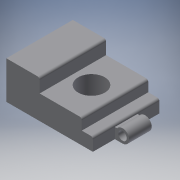
# Autodesk Inventor part: Hinge, Explosion Button
Saved by Autodesk Inventor 2016 (Build 200138000, 138)
## iProperties
Created: 2016-03-16
Part Number: Hinge, Explosion Button
Material: Generic
Document SubType Name: Modeling
Designer: Owner
Density: 1 g/cm^3
Appearance: Default
Author: Owner
Autodesk Inventor part; units mm, degrees
ref_plane "YZ Plane" through (0, 0, 0) normal (1, 0, 0) x (0, 1, 0)
sketch "Sketch1" plane through (0, 0, 0) normal (0, 0, 1) x (1, 0, 0)
  line L0 (0, 0) -> (3.81, 0)
  line L1 (0, 0) -> (0, 1.27)
  arc A0 (3.81, 0) -> (1.359061, 1.27) centre (3.81, 3) ccw
  circle A1 centre (3.81, 3) radius 1.9
  line L2 (0, 1.27) -> (1.359061, 1.27)
  dimension "d0" = 3.81
  dimension "d1" = 1.27
  dimension "d2" = 6
  dimension "d3" = 3.8
  constraints: 6 end point, 2 centre point, 2 point on circle, 1 coincident, 1 horizontal, 1 perpendicular, 1 tangent, 1 vertical
  measures "d0" distance of L0.start L0.end
  measures "d1" distance of L0.start L1.end
  measures "d2" diameter of A0
  measures "d3" diameter of A1
extrude "Extrusion1" add sketch "Sketch1" along normal blind 30.48
ref_plane "Work Plane1" through (0, 0, 20.32) normal (0, 0, 1) x (1, 0, 0)
sketch "Sketch2" plane through (0, 0, 20.32) normal (0, 0, 1) x (1, 0, 0)
  arc A0 (3.81, 0) -> (1.359061, 1.27) centre (3.81, 3) ccw
  line L0 (2.54, 1.27) -> (2.54, 0)
  line L1 (0, 0) -> (3.81, 0)
  line L2 (2.54, 0) -> (3.81, 0)
  circle A1 centre (3.81, 3) radius 0.762
  constraints: 4 end point, 1 centre point, 1 coincident, 1 horizontal, 1 point on line, 1 tangent, 1 vertical, 1 other
sketch "Sketch2 outline for Extrusion5" plane through (0, 0, 20.32) normal (0, 0, 1) x (1, 0, 0)
  line L0 (2.54, 0) -> (3.81, 0)
  line L1 (1.359061, 1.27) -> (2.54, 0)
  arc A0 (3.81, 0) -> (1.359061, 1.27) centre (3.81, 3) ccw
  circle A1 centre (3.81, 3) radius 0.762
extrude "Extrusion5" cut sketch "Sketch2 outline for Extrusion5" along normal blind 25.4
ref_plane "Work Plane3" through (0, 0, 10.16) normal (0, 0, -1) x (-1, 0, 0)
sketch "Sketch6" plane through (0, 0, 10.16) normal (0, 0, -1) x (-1, 0, 0)
  line L0 (-1.359061, 1.27) -> (-2.54, 0)
  line L1 (-1.359061, 1.27) -> (-2.54, 0)
  circle A0 centre (-3.81, 1.27) radius 0.762
  arc A1 (-1.359061, 1.27) -> (-3.81, 0) centre (-3.81, 3) ccw
  line L2 (-2.54, 0) -> (-3.81, 0)
  point P0 (0, 0)
  constraints: 4 end point, 1 centre point, 1 collinear, 1 horizontal, 1 tangent
extrude "Extrusion6" cut sketch "Sketch6" along normal blind 25.4
sketch "Sketch8" plane through (0, 0, 30.48) normal (0, 0, 1) x (1, 0, 0)
  line L0 (1.633512, 1.27) -> (1.633512, 0)
  line L1 (1.633512, 1.27) -> (1.633512, 0)
  line L2 (1.359061, 1.27) -> (2.54, 0)
  line L3 (1.633512, 0) -> (2.54, 0)
  line L4 (1.359061, 1.27) -> (0, 1.27)
  line L5 (2.54, 0) -> (1.633512, 1.27)
  point P0 (0, 0)
  constraints: 6 end point, 1 perpendicular, 1 vertical, 2 other
extrude "Extrusion8" cut sketch "Sketch8" against normal blind 10.16
sketch "Sketch9" plane through (0, 0, 0) normal (0, 0, -1) x (-1, 0, 0)
  arc A0 (-4.571927, 1.259464) -> (-3.048073, 1.259464) centre (-3.81, 1.27) ccw
  arc A1 (-4.571927, 1.259464) -> (-3.048073, 1.259464) centre (-3.81, 3) ccw
  point P0 (0, 0)
extrude "Extrusion9" cut sketch "Sketch9" against normal blind 10.16
sketch "Sketch10" plane through (0, 0, 0) normal (0, 0, -1) x (-1, 0, 0)
  line L0 (-1.359061, 1.27) -> (0, 1.27)
  line L1 (-1.359061, 1.27) -> (-1.359061, 0)
  line L2 (-1.359061, 0) -> (-2.542741, 0)
  line L3 (-2.542741, 0) -> (-1.359061, 1.27)
  point P0 (0, 0)
  constraints: 6 end point, 1 perpendicular, 1 vertical
extrude "Extrusion10" cut sketch "Sketch10" against normal blind 10.16
sketch "Sketch11" plane through (0, 0, 30.48) normal (0, 0, 1) x (1, 0, 0)
  line L0 (1.359061, 1.27) -> (1.633512, 1.27)
  line L1 (1.359061, 1.27) -> (1.633512, 0.974851)
  line L2 (1.633512, 1.27) -> (1.633512, 0.974851)
  line L3 (1.633512, 0.974851) -> (1.359061, 1.27)
  point P0 (0, 0)
  constraints: 6 end point, 1 collinear, 1 horizontal, 1 perpendicular
extrude "Extrusion11" add sketch "Sketch11" against normal blind 10.16
sketch "Sketch12" plane through (0, 1.27, 30.48) normal (0, 1, 0) x (1, 0, 0)
  line L0 (1.359061, 30.48) -> (1.359061, 20.32)
  line L1 (1.359061, 30.48) -> (-8.640939, 30.48)
  line L2 (-8.640939, 30.48) -> (-8.640939, 0)
  line L3 (-8.640939, 0) -> (1.359061, 0)
  line L4 (1.359061, 0) -> (1.359061, 30.48)
  point P0 (0, 30.48)
  dimension "d34" = 10
  constraints: 8 end point, 2 parallel, 1 horizontal, 1 perpendicular
  measures "d34" distance of L2.end L3.end
extrude "Extrusion12" add sketch "Sketch12" against normal blind 1.27
sketch "Sketch13" plane through (1.633512, 1.27, 30.48) normal (0, 1, 0) x (1, 0, 0)
  line L0 (-0.274451, 30.48) -> (-0.274451, 20.32)
  line L1 (-0.274451, 20.32) -> (-0.274451, 0)
  line L2 (-0.274451, 0) -> (1.648434, 0)
  line L3 (1.648434, 0) -> (1.648434, 10.16)
  line L4 (2.176488, 10.16) -> (0, 10.16)
  line L5 (-0.274451, 10.16) -> (1.648434, 10.16)
  point P0 (-1.633512, 30.48)
  constraints: 8 end point, 3 perpendicular, 1 midpoint, 1 point on line, 1 vertical
extrude "Extrusion13" cut sketch "Sketch13" against normal blind 1.27
sketch "Sketch14" plane through (1.359061, 0, 0) normal (1, 0, 0) x (0, 0, -1)
  line L0 (-30.474923, 6.35) -> (0.005077, 6.35)
  line L1 (0.005077, 6.35) -> (0.005077, 0)
  line L2 (0, 1.27) -> (-30.48, 1.27)
  line L3 (0, 1.27) -> (-30.474923, 1.27)
  line L4 (-30.474923, 1.27) -> (-30.474923, 5.77)
  line L5 (-30.474923, 5.77) -> (0, 5.77)
  line L6 (0, 5.77) -> (0, 1.27)
  point P0 (0, 0)
  dimension "d39" = 4.5
  constraints: 8 end point, 2 parallel, 1 horizontal, 1 perpendicular
  measures "d39" distance of L5.end L2.start
extrude "Extrusion14" add sketch "Sketch14" against normal blind 10
sketch "Sketch15" plane through (1.359061, 0, 20.32) normal (1, 0, 0) x (0, 0, -1)
  line L0 (-10.154923, 5.77) -> (20.32, 5.77)
  line L1 (20.32, 0) -> (20.07, 0)
  line L2 (20.07, 0) -> (20.07, 5.77)
  line L3 (20.07, 5.77) -> (20.32, 5.77)
  line L4 (20.32, 5.77) -> (20.32, 0)
  line L5 (-10.154923, 5.77) -> (20.32, 5.77)
  line L6 (5.082538, 5.77) -> (5.082538, 11.076995)
  line L7 (-10.154923, 0) -> (-9.904923, 0)
  line L8 (-9.904923, 0) -> (-9.904923, 5.77)
  line L9 (-10.154923, 5.77) -> (-10.154923, 0)
  line L10 (-10.154923, 0) -> (-9.904923, 0)
  line L11 (-9.904923, 0) -> (-9.904923, 5.77)
  line L12 (-9.904923, 5.77) -> (-10.154923, 5.77)
  line L13 (-10.154923, 5.77) -> (-10.154923, 0)
  dimension "d42" = 0.25
  constraints: 24 end point, 4 parallel, 4 symmetric about line, 2 horizontal, 2 perpendicular, 1 midpoint, 1 point on line, 1 vertical
  measures "d42" distance of L1.start L1.end
extrude "Extrusion15" cut sketch "Sketch15" against normal blind 10
sketch "Sketch16" plane through (1.359061, 0, 30.474923) normal (0, 0, -1) x (-1, 0, 0)
  line L0 (0, 1.27) -> (10, 1.27) projected
  line L1 (0, 0) -> (0, 1.27) projected
  line L2 (10, 0) -> (0, 0) projected
  line L3 (10, 1.27) -> (10, 0) projected
  point P0 (1.359061, 0)
extrude "Extrusion16" cut sketch "Sketch16" against normal blind 10
sketch "Sketch17" plane through (1.359061, 5.77, 30.224923) normal (0, 1, 0) x (1, 0, 0)
  line L0 (-5, 33.422895) -> (-5, -3.422186)
  line L1 (0, 29.974923) -> (-10, 29.974923)
  line L2 (-10, 0) -> (-10, 29.974923)
  line L3 (-5, 29.974923) -> (-10, 29.974923)
  line L4 (-10, 29.974923) -> (-10, 0)
  line L5 (-10, 0) -> (-5, 0)
  line L6 (-5, 0) -> (-5, 29.974923)
  point P0 (-1.359061, 30.224923)
  constraints: 8 end point, 2 parallel, 1 horizontal, 1 midpoint, 1 perpendicular
extrude "Extrusion17" add sketch "Sketch17" along normal blind 5
sketch "Sketch18" plane through (1.359061, 0, 0.25) normal (0, 0, -1) x (-1, 0, 0)
  line L0 (40, 0) -> (40, 21.034494)
  line L1 (40, 37.49) -> (40, 17.49)
  line L2 (10, 10.77) -> (5, 10.77)
  line L3 (10, 10.77) -> (40, 10.77)
  line L4 (40, 10.77) -> (40, 0)
  line L5 (40, 0) -> (10, 0)
  line L6 (10, 0) -> (10, 10.77)
  line L7 (25, 10.77) -> (40, 10.77)
  line L8 (40, 10.77) -> (40, 17.49)
  line L9 (40, 17.49) -> (25, 17.49)
  line L10 (25, 17.49) -> (25, 10.77)
  point P0 (1.359061, 0)
  constraints: 16 end point, 4 parallel, 2 horizontal, 2 perpendicular, 1 midpoint
extrude "Extrusion18" add sketch "Sketch18" against normal blind 29.975
sketch "Sketch19" plane through (1.359061, 10.77, 30.224923) normal (0, 1, 0) x (1, 0, 0)
  circle A0 centre (-16.625, 15.003923) radius 6
  circle A1 centre (-16.625, 15.003923) radius 4.85
  point P0 (-1.359061, 30.224923)
  dimension "d51" = 12
  constraints: 1 centre point
  measures "d51" diameter of A0
extrude "Extrusion19" cut sketch "Sketch19" against normal blind 29.975 contours A0 | A1
sketch "Sketch20" plane through (1.359061, 0, 30.225) normal (0, 0, 1) x (1, 0, 0)
  line L0 (-25, 17.49) -> (-25, 10.77) projected
  line L1 (-40, 0) -> (-40, 17.49) projected
  line L2 (-25, 17.49) -> (-40, 17.49)
  line L3 (-40, 17.49) -> (-40, 16.99)
  line L4 (-40, 16.99) -> (-25, 16.99)
  line L5 (-25, 16.99) -> (-25, 17.49)
  point P0 (-1.359061, 0)
  dimension "d54" = 0.5
  constraints: 8 end point, 2 parallel, 1 horizontal, 1 perpendicular, 1 point on line
  measures "d54" distance between parallel lines of L4 L2
extrude "Extrusion20" cut sketch "Sketch20" against normal blind 584.2
sketch "Sketch21" plane through (1.359061, 0, 20.32) normal (1, 0, 0) x (0, 0, -1)
  line L0 (20.07, 0) -> (20.07, 5.77)
  line L1 (-9.904923, 5.77) -> (20.07, 5.77)
  line L2 (-9.904923, 5.77) -> (-9.904923, 0)
  line L3 (0, 0) -> (-9.904923, 0)
  line L4 (0, 4.73) -> (0, 0)
  line L5 (10.16, 4.73) -> (0, 4.73)
  line L6 (10.16, 0) -> (10.16, 4.73)
  line L7 (20.07, 0) -> (10.16, 0)
  point P0 (20.32, 0)
extrude "Extrusion21" cut sketch "Sketch21" against normal blind 1
sketch "Sketch22" plane through (-3.640939, 5.77, 30.224923) normal (1, 0, 0) x (0, 0, -1)
  line L0 (0, 0) -> (0, 5)
  line L1 (0, 5) -> (29.974923, 5)
  line L2 (29.974923, 0) -> (29.974923, 5)
  line L3 (29.974923, 0) -> (0, 0)
  point P0 (30.224923, -5.77)
extrude "Extrusion22" cut sketch "Sketch22" against normal blind 1
fillet "Fillet1" radius 1 3 edges at (-23.6409, 16.99, 15.2375) (-4.6409, 10.77, 15.2375) (0.3591, 5.77, 15.2375)
sketch "Sketch23" plane through (1.359061, 0, 30.225) normal (0, 0, 1) x (1, 0, 0)
  spline S0 degree 3 poles (-15.287382, 7.562173) (-14.295298, 10.29556) (-13.653422, 13.152751) (-13.101138, 18.99204) (-13.207044, 21.960303) (-14.220005, 28.120528) (-15.237278, 31.317012) (-16.686921, 34.297861) knots -3.03465801 -3.03465801 -3.03465801 -3.03465801 -2.16997566 -2.16997566 -1.29383861 -1.29383861 -0.2991038 -0.2991038 -0.2991038 -0.2991038
  arc A0 (-25, 15.99) -> (-26, 16.99) centre (-26, 15.99) ccw
  line L0 (-26, 16.99) -> (-40, 16.99)
  line L1 (-40, 16.99) -> (-40, 0)
  line L2 (-40, 0) -> (-10, 0)
  line L3 (-10, 0) -> (-10, 10.77)
  line L4 (-10, 10.77) -> (-25, 10.77)
  line L5 (-25, 10.77) -> (-25, 15.99)
  arc A1 (-1, 4.77) -> (-2, 5.77) centre (-2, 4.77) ccw
  line L6 (-6, 5.77) -> (-2, 5.77)
  line L7 (-6, 5.77) -> (-6, 9.77)
  arc A2 (-6, 9.77) -> (-7, 10.77) centre (-7, 9.77) ccw
  line L8 (-10, 10.77) -> (-7, 10.77)
  line L9 (-10, 0) -> (-10, 10.77)
  line L10 (-1, 0) -> (-10, 0)
  line L11 (-1, 0) -> (-1, 4.77)
  point P0 (-1.359061, 0)
extrude "Extrusion23" add sketch "Sketch23" against normal blind 0.025
sketch "Sketch24" plane through (-38.640939, 0, 0.25) normal (0, 0, -1) x (-1, 0, 0)
  arc A0 (-38, 5.77) -> (-39, 4.77) centre (-38, 4.77) ccw projected
  line L0 (-39, 4.77) -> (-39, 0) projected
  line L1 (-39, 0) -> (0, 0) projected
  line L2 (0, 0) -> (0, 16.99) projected
  line L3 (0, 16.99) -> (-14, 16.99) projected
  arc A1 (-14, 16.99) -> (-15, 15.99) centre (-14, 15.99) ccw projected
  line L4 (-15, 15.99) -> (-15, 10.77) projected
  line L5 (-33, 10.77) -> (-15, 10.77) projected
  arc A2 (-33, 10.77) -> (-34, 9.77) centre (-33, 9.77) ccw projected
  line L6 (-34, 9.77) -> (-34, 5.77) projected
  line L7 (-38, 5.77) -> (-34, 5.77) projected
  point P0 (-38.640939, 0)
extrude "Extrusion24" cut sketch "Sketch24" against normal blind 0.025
body "Solid1"
